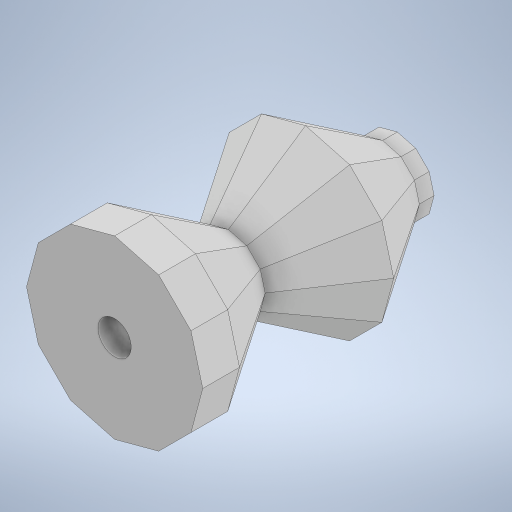
# Autodesk Inventor part: Test21
Saved by Autodesk Inventor 2023 (Build 270158000, 158)
## iProperties
Created: 2024-07-02
Part Number: Test21
Material: 일반
Document SubType Name: Modeling
Designer: ojs08
Density: 1 g/cm^3
Appearance: 기본값
Author: ojs08
Autodesk Inventor part; units mm, degrees
ref_plane "YZ Plane" through (0, 0, 0) normal (1, 0, 0) x (0, 1, 0)
ref_plane "XZ Plane" through (0, 0, 0) normal (0, 1, 0) x (-1, 0, 0)
sketch "스케치1" plane through (0, 0, 0) normal (0, 0, 1) x (1, 0, 0)
  line L0 (12, 0) -> (10.3923, -6)
  line L1 (10.3923, -6) -> (6, -10.3923)
  line L2 (6, -10.3923) -> (0, -12)
  line L3 (0, -12) -> (-6, -10.3923)
  line L4 (-6, -10.3923) -> (-10.3923, -6)
  line L5 (-10.3923, -6) -> (-12, 0)
  line L6 (-12, 0) -> (-10.3923, 6)
  line L7 (-10.3923, 6) -> (-6, 10.3923)
  line L8 (-6, 10.3923) -> (0, 12)
  line L9 (0, 12) -> (6, 10.3923)
  line L10 (6, 10.3923) -> (10.3923, 6)
  line L11 (10.3923, 6) -> (12, 0)
  line L12 (-16.8, 0) -> (16.8, 0) projected
  point P0 (0, 0)
  dimension "d1" = 24
  constraints: 24 end point, 1 point on line, 25 other
  measures "d1" distance of L0.start L5.end
ref_plane "작업 평면1" through (0, 0, 10.5) normal (0, 0, 1) x (1, 0, 0)
sketch "스케치2" plane through (0, 0, 10.5) normal (0, 0, 1) x (1, 0, 0)
  line L0 (4.3301, -2.5) -> (2.5, -4.3301)
  line L1 (2.5, -4.3301) -> (0, -5)
  line L2 (0, -5) -> (-2.5, -4.3301)
  line L3 (-2.5, -4.3301) -> (-4.3301, -2.5)
  line L4 (-4.3301, -2.5) -> (-5, 0)
  line L5 (-5, 0) -> (-4.3301, 2.5)
  line L6 (-4.3301, 2.5) -> (-2.5, 4.3301)
  line L7 (-2.5, 4.3301) -> (0, 5)
  line L8 (0, 5) -> (2.5, 4.3301)
  line L9 (2.5, 4.3301) -> (4.3301, 2.5)
  line L10 (4.3301, 2.5) -> (5, 0)
  line L11 (5, 0) -> (4.3301, -2.5)
  line L12 (-16.8, 0) -> (16.8, 0) projected
  point P0 (0, 0)
  point P1 (0, 0)
  dimension "d4" = 10
  constraints: 24 end point, 1 coincident, 1 point on line, 25 other
  measures "d4" distance of L10.end L4.end
loft "로프트1" add profiles "스케치1", "스케치2"
mirror "미러1" about plane through (0, 0, 10.5) normal (0, 0, 1) of "로프트1"
mirror "미러2" about plane through (0, 0, 0) normal (0, 0, -1) of "로프트1"
sketch "스케치3" plane through (10.3923, -6, 21) normal (0, 0, 1) x (0.9659258, -0.258819, 0)
  line L0 (0, 6.2117) -> (0, 0) projected
  line L1 (-3.1058, 11.5911) -> (0, 6.2117) projected
  line L2 (-8.4853, 14.6969) -> (-3.1058, 11.5911) projected
  line L3 (-14.6969, 14.6969) -> (-8.4853, 14.6969) projected
  line L4 (-20.0764, 11.5911) -> (-14.6969, 14.6969) projected
  line L5 (-23.1822, 6.2117) -> (-20.0764, 11.5911) projected
  line L6 (-23.1822, 0) -> (-23.1822, 6.2117) projected
  line L7 (-20.0764, -5.3795) -> (-23.1822, 0) projected
  line L8 (-14.6969, -8.4853) -> (-20.0764, -5.3795) projected
  line L9 (-8.4853, -8.4853) -> (-14.6969, -8.4853) projected
  line L10 (-3.1058, -5.3795) -> (-8.4853, -8.4853) projected
  line L11 (0, 0) -> (-3.1058, -5.3795) projected
  point P0 (-11.5911, 3.1058)
extrude "돌출1" add sketch "스케치3" along normal blind 2
shell "쉘1" thickness 0.5 removed faces 0 ; own thickness 2 on faces at (2.7083, 10.1076, -1.75) (7.3993, 7.3993, -1.75) (10.1076, 2.7083, -1.75) (10.1076, -2.7083, -1.75) (7.3993, -7.3993, -1.75) (2.7083, -10.1076, -1.75) (-2.7083, -10.1076, -1.75) (-2.7083, 10.1076, -1.75) (-7.3993, 7.3993, -1.75) (-10.1076, 2.7083, -1.75) (-10.1076, -2.7083, -1.75) (-7.3993, -7.3993, -1.75) (2.7083, -10.1076, 19.25) (7.3993, -7.3993, 19.25) (10.1076, -2.7083, 19.25) (10.1076, 2.7083, 19.25) (-2.7083, -10.1076, 19.25) (-7.3993, -7.3993, 19.25) (-10.1076, -2.7083, 19.25) (-10.1076, 2.7083, 19.25) (-7.3993, 7.3993, 19.25) (7.3993, 7.3993, 19.25) (2.7083, 10.1076, 19.25) (-2.7083, 10.1076, 19.25)
sketch "스케치4" plane through (10.3923, -6, 23) normal (0, 0, 1) x (0.9659258, -0.258819, 0)
  line L0 (-3.1058, 11.5911) -> (-8.4853, 14.6969) projected
  line L1 (-8.4853, 14.6969) -> (-14.6969, 14.6969) projected
  line L2 (-14.6969, 14.6969) -> (-20.0764, 11.5911) projected
  line L3 (-20.0764, 11.5911) -> (-23.1822, 6.2117) projected
  line L4 (-23.1822, 6.2117) -> (-23.1822, 0) projected
  line L5 (-23.1822, 0) -> (-20.0764, -5.3795) projected
  line L6 (-20.0764, -5.3795) -> (-14.6969, -8.4853) projected
  line L7 (-14.6969, -8.4853) -> (-8.4853, -8.4853) projected
  line L8 (-8.4853, -8.4853) -> (-3.1058, -5.3795) projected
  line L9 (-3.1058, -5.3795) -> (0, 0) projected
  line L10 (0, 0) -> (0, 6.2117) projected
  line L11 (0, 6.2117) -> (-3.1058, 11.5911) projected
  point P0 (-11.5911, 3.1058)
extrude "돌출2" add sketch "스케치4" along normal blind 3
sketch "스케치5" plane through (10.3923, -6, 26) normal (0, 0, 1) x (0.9659258, -0.258819, 0)
  circle A0 centre (-11.5911, 3.1058) radius 2.25
  dimension "d15" = 4.5
  constraints: 1 centre point, 1 coincident
  measures "d15" diameter of A0
extrude "돌출3" cut sketch "스케치5" against normal blind 5
sketch "스케치6" plane through (4.3301, -2.5, -10.5) normal (0, 0, -1) x (-0.9659258, 0.258819, 0)
  line L0 (0, 2.5882) -> (0, 0) projected
  line L1 (0, 0) -> (1.2941, -2.2414) projected
  line L2 (1.2941, -2.2414) -> (3.5355, -3.5355) projected
  line L3 (3.5355, -3.5355) -> (6.1237, -3.5355) projected
  line L4 (6.1237, -3.5355) -> (8.3652, -2.2414) projected
  line L5 (8.3652, -2.2414) -> (9.6593, 0) projected
  line L6 (9.6593, 0) -> (9.6593, 2.5882) projected
  line L7 (9.6593, 2.5882) -> (8.3652, 4.8296) projected
  line L8 (8.3652, 4.8296) -> (6.1237, 6.1237) projected
  line L9 (6.1237, 6.1237) -> (3.5355, 6.1237) projected
  line L10 (3.5355, 6.1237) -> (1.2941, 4.8296) projected
  line L11 (1.2941, 4.8296) -> (0, 2.5882) projected
  point P0 (4.8296, 1.2941)
extrude "돌출4" add sketch "스케치6" along normal blind 2
